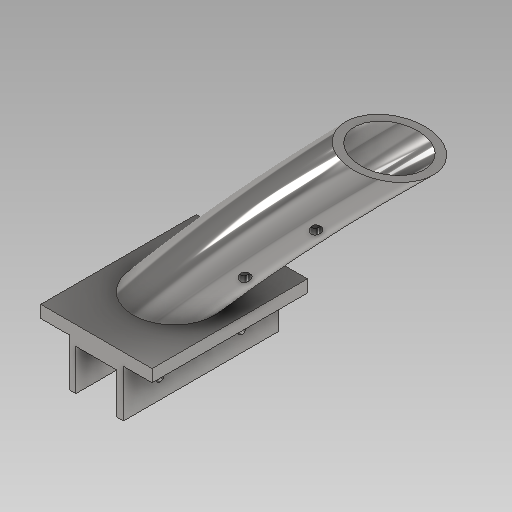
# Autodesk Inventor part: support_basePart
Saved by Autodesk Inventor 2021 (Build 250183000, 183)
## iProperties
Created: 2021-05-24
Part Number: support_basePart
Material: Steel, High Strength, Low Alloy
Document SubType Name: Modeling
Designer: Watchdog
Density: 7.85 g/cm^3
Appearance: Steel - Polished
Author: Watchdog
Autodesk Inventor part; units mm, degrees
ref_plane "YZ Plane" through (0, 0, 0) normal (1, 0, 0) x (0, 1, 0)
ref_plane "XZ Plane" through (0, 0, 0) normal (0, 1, 0) x (-1, 0, 0)
ref_plane "XY Plane" through (0, 0, 0) normal (0, 0, 1) x (1, 0, 0)
sketch "Sketch1" plane through (0, 0, 0) normal (0, 0, 1) x (1, 0, 0)
  line L0 (-33, 0) -> (33, 0)
  line L1 (33, 0) -> (33, -58)
  line L2 (33, -58) -> (-33, -58)
  line L3 (-33, -58) -> (-33, 0)
  point P0 (0, 0)
  dimension "d0" = 58
  dimension "d1" = 66
  dimension "d2" = 33
  dimension "d3" = 0
  constraints: 8 end point, 2 parallel, 1 horizontal, 1 perpendicular
  measures "d0" distance of L2.end L0.start
  measures "d1" distance of L0.start L0.end
  measures "d2" distance from line of point (0, 0) L3
  measures "d3" distance from line of point (0, 0) L0
extrude "clamp_base" add sketch "Sketch1" against normal blind 190
sketch "Sketch2" plane through (0, 0, 0) normal (0, 0, 1) x (1, 0, 0)
  line L0 (-25, -58) -> (25, -58)
  line L1 (25, -58) -> (25, -8)
  line L2 (25, -8) -> (-25, -8)
  line L3 (-25, -8) -> (-25, -58)
  line L4 (-33, -58) -> (33, -58) projected
  point P0 (0, 0)
  dimension "d6" = 50
  dimension "d7" = 50
  dimension "d8" = 25
  constraints: 8 end point, 2 parallel, 1 collinear, 1 horizontal, 1 perpendicular
  measures "d6" distance between parallel lines of L1 L3
  measures "d7" distance of L2.end L0.start
  measures "d8" distance from line of point (0, 0) L3
extrude "clamp_extrusion" cut sketch "Sketch2" against normal through all
sketch "Sketch4" plane through (-33, 0, 0) normal (0, 1, 0) x (1, 0, 0)
  line L0 (-35, 190) -> (101, 190)
  line L1 (101, 190) -> (101, 0)
  line L2 (101, 0) -> (-35, 0)
  line L3 (-35, 0) -> (-35, 190)
  line L4 (66, 0) -> (0, 0) projected
  line L5 (0, 190) -> (66, 190) projected
  line L6 (0, 0) -> (0, 190) projected
  line L7 (66, 0) -> (66, 190) projected
  point P0 (33, 0)
  dimension "d35" = 0
  dimension "d36" = 0
  dimension "d37" = 35
  dimension "d38" = 35
  constraints: 8 end point, 2 parallel, 1 horizontal, 1 perpendicular
  measures "d35" distance between parallel lines of L2 L4
  measures "d36" distance between parallel lines of L0 L5
  measures "d37" distance between parallel lines of L6 L3
  measures "d38" distance between parallel lines of L1 L7
extrude "platform" add sketch "Sketch4" along normal blind 15
sketch "Sketch5" plane through (-33, 15, 0) normal (0, 1, 0) x (1, 0, 0)
  circle A0 centre (33, 95) radius 40
  circle A1 centre (33, 95) radius 50
  line L0 (101, 190) -> (-35, 190) projected
  line L1 (-35, 0) -> (101, 0) projected
  point P0 (33, 0)
  dimension "d15" = 80
  dimension "d16" = 0
  dimension "d17" = 95
  dimension "d20" = 100
  dimension "d62" = 190
  constraints: 2 centre point, 2 coincident
  measures "d15" diameter of A0
  measures "d16" horizontal distance of point (33, 0) A0.centre
  measures "d17" distance of point (33, 0) A0.centre
  measures "d20" diameter of A1
  measures "d62" distance between parallel lines of L0 L1
ref_plane "align_sleeve" through (0, 15, -95) normal (-0.7071068, 0, -0.7071068) x (0, 1, 0)
ref_plane "hoop_zAngle" through (68, 0, -190) normal (-0.7071068, 0, -0.7071068) x (0, 1, 0)
sketch "Sketch6" plane through (0, 15, -95) normal (-0.7071068, 0, -0.7071068) x (0, 1, 0)
  line L0 (0, -19.0919) -> (0, 115.2584) projected
  arc A0 (0, 0) -> (151.6009, 186.074) centre (-1200, 1132.4752) ccw
  line L1 (-1200, 1132.4752) -> (438.3041, -14.6777)
  line L2 (54.0581, 1398.7763) -> (54.0581, 1220.5849)
  point P0 (-15, -67.1751)
  dimension "d28" = 1200
  dimension "d29" = 1650
  dimension "d31" = 55
  dimension "d32" = 2000
  constraints: 4 end point, 2 point on circle, 1 centre point, 1 point on line, 1 vertical
  measures "d28" distance from line of L0 L1.start
  measures "d29" radius of A0
  measures "d31" angle of L2 L1
  measures "d32" distance of L1.start L1.end
sweep "sleeve" add profiles "Sketch5" path "Sketch6" path curves A0
ref_plane "align_hole" through (-19.7904, 35.3982, -145.9203) normal (-0.7071068, 0, -0.7071068) x (0, -1, 0)
sketch "Sketch7" plane through (-19.7904, 35.3982, -145.9203) normal (-0.7071068, 0, -0.7071068) x (0, -1, 0)
  line L0 (20.3982, -27.9879) -> (20.3982, 72.0121) projected
  arc A0 (20.3982, -13.3432) -> (-126.0734, -199.0432) centre (1220.3982, -1110.463) ccw projected
  line L1 (-138.4565, -114.5909) -> (-123.9488, -213.5329) projected
  line L2 (-134.3557, -117.932) -> (20.3982, 72.0121)
  line L3 (-128.0496, -210.1919) -> (20.3982, -27.9879)
  point P0 (35.3982, 89.1873)
  point P1 (-79.6018, -100.7273)
  point P2 (-29.6018, -39.3576)
  dimension "d39" = 63.1635
  dimension "d40" = 31.5818
  dimension "d41" = 31.5818
  dimension "d42" = 50
  dimension "d43" = 100
  constraints: 4 end point, 1 parallel
  measures "d39" distance between parallel lines of L3 L2
  measures "d40" distance from line of point (-79.602, -100.727) L2
  measures "d41" distance from line of L2 point (-29.602, -39.358)
  measures "d42" distance from line of L0 point (-29.602, -39.358)
  measures "d43" distance from line of L0 point (-79.602, -100.727)
hole "sleeveHole" at (51.4345, 115, -217.1452) at (8.0396, 65, -173.7503) direction (0.7071068, 0, 0.7071068) diameter 12 end through all
sketch "Sketch8" plane through (33, -58, 0) normal (1, 0, 0) x (0, 0, -1)
  line L0 (0, 0) -> (0, 58) projected
  line L1 (190, 58) -> (190, 0) projected
  point P0 (45, 24.0271)
  point P1 (145, 24.0271)
  dimension "d51" = 45
  dimension "d60" = 100
  dimension "d61" = 190
  measures "d51" distance from line of L0 point (45, 24.027)
  measures "d60" distance of point (145, 24.027) point (45, 24.027)
  measures "d61" distance between parallel lines of L1 L0
hole "clampHole" at (33, -33.9729, -45) at (33, -33.9729, -145) direction (-1, 0, 0) diameter 10 end through all
equation "\"d0\" = support_frame_squareBarDimension + support_baseClamp_thickness"
equation "\"d1\" = support_frame_squareBarDimension + 2 * support_baseClamp_thickness"
equation "\"d2\" = 0.5 * d1"
equation "\"d4\" = width"
equation "\"d6\" = support_frame_squareBarDimension"
equation "\"d7\" = support_frame_squareBarDimension"
equation "\"d8\" = 0.5 * d6"
equation "\"d37\" = support_baseClamp_platformLengthBuffer"
equation "\"d38\" = support_baseClamp_platformLengthBuffer"
equation "\"d13\" = support_baseClamp_platformThickness"
equation "\"d15\" = hoop_width_large"
equation "\"d17\" = 0.5 * d62"
equation "\"d20\" = hoop_width_large + sleeveThickness"
equation "\"d28\" = r - y"
equation "\"d29\" = r"
equation "\"d31\" = phi"
equation "\"d40\" = 0.5 * d39"
equation "\"d41\" = d40"
equation "\"d42\" = support_baseClamp_sleeve_hole1Height"
equation "\"d43\" = support_baseClamp_sleeve_hole2Height"
equation "\"d44\" = sleeveHoleDiameter"
equation "\"d51\" = -0.5 * d60 + 0.5 * d61"
equation "\"d60\" = clampHoleSpacing"
equation "\"d53\" = clampHoleDiameter"
equation "\"hoop_width_large\" = 80"
equation "\"width\" = clampHoleDiameter + clampHoleSpacing + 2 * buffer"
equation "\"clampHoleSpacing\" = support_frame_clampHoleSpacing"
equation "\"clampHoleDiameter\" = support_frame_clampHoleDiameter"
equation "\"sleeveThickness\" = support_baseClamp_sleeveThickness"
equation "\"d26\" = theta"
equation "\"sleeveHoleDiameter\" = support_baseClamp_sleeveHoleDiameter"
equation "\"y\" = hoop_height_large"
equation "\"r\" = 0.5 * hoop_radius_large"
equation "\"theta\" = hoop_angle_z"
equation "\"phi\" = support_baseClamp_sleeveSweepTerminationAngle"
equation "\"support_frame_squareBarDimension\" = 50"
equation "\"support_baseClamp_thickness\" = 8"
equation "\"support_baseClamp_sleeveHoleDiameter\" = 12"
equation "\"hoop_angle_z\" = 45deg"
equation "\"support_baseClamp_sleeveSweepTerminationAngle\" = 55deg"
equation "\"support_baseClamp_platformThickness\" = 15"
equation "\"support_baseClamp_platformWidthBuffer\" = 0"
equation "\"support_baseClamp_platformLengthBuffer\" = 35"
equation "\"rack_tooth_thickness\" = 5"
equation "\"rack_tooth_addendum\" = 5"
equation "\"rack_tooth_dedendum\" = 5"
equation "\"hoop_bearing_length\" = 5deg"
equation "\"hoop_cable_diam\" = 5"
equation "\"hoop_cable_pulley_diam\" = 22"
equation "\"secure_arm_radii\" = 9"
equation "\"secure_arm_hold_length\" = 35"
equation "\"secure_arm_angle\" = 20deg"
equation "\"support_frame_endHoleBuffer\" = 25"
equation "\"support_baseClamp_sleeve_hole1Height\" = 50"
equation "\"support_baseClamp_sleeve_hole2Height\" = 100"
equation "\"hoop_tabs_thickness\" = 6"
equation "\"support_frame_squareBarThickness\" = 5"
equation "\"wheelchair_deployed_length\" = 1067"
equation "\"wheelchair_deployed_height\" = 914"
equation "\"hoop_tabs_hole\" = 4"
equation "\"wheelchair_deployed_width\" = 635"
equation "\"support_frame_squareBarFillet\" = 2"
equation "\"buffer\" = 40"
equation "\"support_frame_clampHoleSpacing\" = 100"
equation "\"support_frame_clampHoleDiameter\" = 10"
equation "\"support_baseClamp_sleeveThickness\" = 20"
equation "\"hoop_height_large\" = 450"
equation "\"hoop_radius_large\" = 3300"
body "Solid1"
